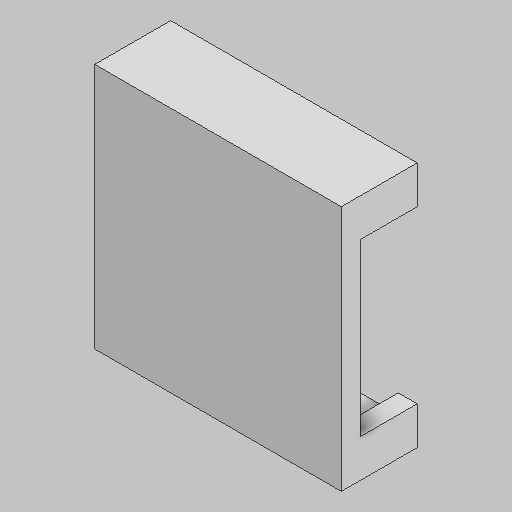
# Autodesk Inventor part: Optical module_lid_2
Saved by Autodesk Inventor 2026.1 (Build 301233020, 233B)
## iProperties
Created: 2026-01-23
Part Number: Optical module_lid_2
Material: Generic
Document SubType Name: Modeling
Designer: samuel
Density: 1 g/cm^3
Appearance: Default
Author: samuel
Autodesk Inventor part; units mm, degrees
ref_plane "YZ Plane" through (0, 0, 0) normal (1, 0, 0) x (0, 1, 0)
ref_plane "XZ Plane" through (0, 0, 0) normal (0, 1, 0) x (-1, 0, 0)
ref_plane "XY Plane" through (0, 0, 0) normal (0, 0, 1) x (1, 0, 0)
sketch "Sketch1" plane through (0, 0, 0) normal (0, 0, 1) x (1, 0, 0)
  line L0 (-6.5, -6.5) -> (6.5, -6.5)
  line L1 (6.5, -6.5) -> (6.5, 6.5)
  line L2 (6.5, 6.5) -> (-6.5, 6.5)
  line L3 (-6.5, 6.5) -> (-6.5, -6.5)
  line L4 (-6.5, -6.5) -> (6.5, 6.5) construction
  line L5 (6.5, -6.5) -> (-6.5, 6.5) construction
  line L6 (-5.5, -5.5) -> (5.5, -5.5)
  line L7 (5.5, -5.5) -> (5.5, 5.5)
  line L8 (5.5, 5.5) -> (-5.5, 5.5)
  line L9 (-5.5, 5.5) -> (-5.5, -5.5)
  line L10 (-5.5, -5.5) -> (5.5, 5.5) construction
  line L11 (5.5, -5.5) -> (-5.5, 5.5) construction
  line L12 (5.5, 5.5) -> (6.5, 5.5)
  line L13 (6.5, 5.5) -> (6.5, 4.5)
  line L14 (6.5, 4.5) -> (5.5, 4.5)
  line L15 (5.5, 4.5) -> (5.5, 5.5)
  line L16 (5.5, -5.5) -> (6.5, -5.5)
  line L17 (6.5, -5.5) -> (6.5, -4.5)
  line L18 (6.5, -4.5) -> (5.5, -4.5)
  line L19 (5.5, -4.5) -> (5.5, -5.5)
  point P0 (0, 0)
  point P1 (5.5, -4.5)
  point P2 (5.5, 4.5)
  dimension "d0" = 13
  dimension "d1" = 13
  dimension "d2" = 11
  dimension "d3" = 11
  dimension "d4" = 1
  dimension "d5" = 1
  constraints: 40 end point, 8 parallel, 4 horizontal, 4 midpoint, 4 perpendicular, 2 point on line
  measures "d0" distance of L2.end L1.end
  measures "d1" distance of L1.end L0.end
  measures "d2" distance of L8.end L7.end
  measures "d3" distance of L7.end L6.end
  measures "d4" distance of L12.end L13.end
  measures "d5" distance of L17.end L16.end
extrude "Extrusion1" add sketch "Sketch1" along normal blind 4
extrude "Extrusion2" cut sketch "Sketch1" along normal blind 2 contours L18 L7 L14 L1 | L6 L9 L8 L7
sketch "Sketch2" plane through (0, 0, 2) normal (0, 0, -1) x (-1, 0, 0)
  line L0 (-6.5, -6.5) -> (-6.5, 6.5) projected
  line L1 (-5.5, -4.5) -> (-6.5, -4.5) projected
  line L2 (-6.5, 4.5) -> (-5.5, 4.5)
  line L3 (-5.5, 4.5) -> (-5.5, -4.5)
  line L4 (-5.5, -4.5) -> (-6.5, -4.5)
  line L5 (-6.5, -4.5) -> (-6.5, 4.5)
  line L6 (-6.5, 4.5) -> (-5.5, 4.5) projected
  line L7 (5.5, 5.5) -> (5.5, -5.5) projected
  line L8 (-5.5, 4.5) -> (5.5, 4.5)
  line L9 (5.5, 4.5) -> (5.5, -4.5)
  line L10 (5.5, -4.5) -> (-5.5, -4.5)
  line L11 (-5.5, -4.5) -> (-5.5, 4.5)
  point P0 (0, 0)
  dimension "d18" = 0
  constraints: 16 end point, 4 parallel, 2 horizontal, 2 perpendicular, 2 point on line
  measures "d18" distance between parallel lines of L6 L2
extrude "Extrusion3" cut sketch "Sketch2" against normal blind 1
sketch "Sketch3" plane through (0, 0, 0) normal (0, 0, -1) x (-1, 0, 0)
  line L0 (6.5, 6.5) -> (6.5, -6.5) projected
  line L1 (5.5, 5.5) -> (5.5, -5.5) projected
  line L2 (6.5, 5.5) -> (5.5, 5.5)
  line L3 (5.5, 5.5) -> (5.5, -5.5)
  line L4 (5.5, -5.5) -> (6.5, -5.5)
  line L5 (6.5, -5.5) -> (6.5, 5.5)
  line L6 (-5.5, 5.5) -> (5.5, 5.5) projected
  point P0 (0, 0)
  point P1 (5.5, 5.5)
  dimension "d15" = 0
  constraints: 8 end point, 2 parallel, 1 horizontal, 1 perpendicular, 1 point on line
  measures "d15" distance between parallel lines of L6 L2
extrude "Extrusion4" cut sketch "Sketch3" against normal blind 2
body "Solid1"
